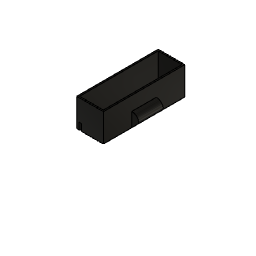
Seitenteil_links_Schublade_v56 (Autodesk Fusion 360 design; units mm, degrees)
Autodesk Fusion 360 part; units mm, degrees
sketch "Skizze1" plane through (70, 0, 0) normal (1, 0, 0) x (0, 1, 0)
  line L0 (59.1546, 143.1) -> (59.1546, 102.1)
  line L1 (59.1546, 102.1) -> (-58.1, 102.1)
  line L2 (-58.1, 102.1) -> (-58.1, 143.1)
  line L3 (-58.1, 143.1) -> (59.1546, 143.1)
  line L4 (-74.1, 83.1) -> (74.1, 83.1)
  line L5 (74.1, 83.1) -> (74.1, 152.2)
  arc A0 (74.1, 152.2) -> (73.2, 153.1) centre (73.2, 152.2) ccw
  line L6 (73.2, 153.1) -> (-73.2, 153.1)
  arc A1 (-73.2, 153.1) -> (-74.1, 152.2) centre (-73.2, 152.2) ccw
  line L7 (-74.1, 152.2) -> (-74.1, 83.1)
  line L8 (-58.1, 102.1) -> (-58.1, 143.1)
  line L9 (-58.1, 143.1) -> (59.1546, 143.1)
  line L10 (59.1546, 143.1) -> (59.1546, 102.1)
  line L11 (59.1546, 102.1) -> (-58.1, 102.1)
  line L12 (-57.6, 142.6) -> (58.6546, 142.6)
  line L13 (58.6546, 142.6) -> (58.6546, 102.6)
  line L14 (58.6546, 102.6) -> (-57.6, 102.6)
  line L15 (-57.6, 102.6) -> (-57.6, 142.6)
  dimension "d664" = 0.5
  dimension "d665" = 0.5
  dimension "d666" = 0.5
  dimension "d667" = 0.5
  constraint horizontal L12
  constraint vertical L13
  constraint horizontal L14
  constraint vertical L15
  measures "d664" distance of L8 L15
  measures "d665" distance of L10 L13
  measures "d666" distance of L9 L12
  measures "d667" distance of L11 L14
extrude "Extrusion1" add sketch "Skizze1" against normal blind 38 contours L12 L13 L14 L15
shell "Schale1" thickness 2 removed faces 1 at (57.3333, -18.8485, 142.6)
sketch "Skizze7" plane through (0, 0, 102.6) normal (0, 0, -1) x (1, 0, 0)
  line L0 (70, -58.6546) -> (70, 57.6)
  line L1 (70, 57.6) -> (32, 57.6)
  line L2 (32, 57.6) -> (32, -58.6546)
  line L3 (32, -58.6546) -> (70, -58.6546)
  circle A0 centre (37, 58.6) radius 2
  circle A1 centre (37, -59.6546) radius 2
  dimension "d728" = 4
  dimension "d730" = 33
  dimension "d731" = 4
  dimension "d749" = 1
  dimension "d750" = 1
  constraint vertical A0.centre A1.centre
  measures "d728" diameter of A0
  measures "d730" distance of L0 A0.centre
  measures "d731" diameter of A1
  measures "d749" distance of L3 A1.centre
  measures "d750" distance of L1 A0.centre
extrude "Extrusion4" cut sketch "Skizze7" against normal up to surface (9.5 mm away) contours L3 A1 | L1 A0 picked at (36.8035, -58.1862) picked at (37.4433, 57.1448)
ref_plane "Arbeitsebene2" through (51, 0.5273, 122.6) normal (0, 1, 0) x (0, 0, -1)
sketch "Skizze4" plane through (51, 0.5273, 124.1) normal (0, 1, 0) x (1, 0, 0)
  arc A0 (19, 1.5) -> (29, 11.5) centre (19, 11.5) ccw
  line L0 (19, -18.5) -> (19, 21.5)
  line L1 (29, 11.5) -> (19, 11.5)
  dimension "d709" = 10
  dimension "d710" = 10
  constraint vertical A0.centre L0.end
  constraint vertical A0.start L0.end
  constraint horizontal A0.centre A0.end
  constraint coincident A0.centre L1.end
  measures "d709" radius of A0
  measures "d710" distance of A0.centre L0.end
extrude "Extrusion2" add sketch "Skizze4" along normal mid plane 35
chamfer "Fase2" distance 10 angle 45 1 edges at (70, 0.5273, 112.6)
sketch "Skizze6" plane through (51, 0.5273, 124.1) normal (0, 1, 0) x (1, 0, 0)
  arc A0 (19, 1.5) -> (29, 11.5) centre (19, 11.5) ccw
  line L0 (19, 21.5) -> (19, 1.5)
  arc A1 (19, 1.5) -> (29, 11.5) centre (19, 11.5) ccw
  line L1 (19, -28.1) -> (19, 41)
  arc A2 (19, 3) -> (27.5, 11.5) centre (18.3872, 12.1128) ccw
  line L2 (19, 3) -> (19, 11.5)
  line L3 (29, 11.5) -> (19, 21.5)
  line L4 (27.5, 11.5) -> (29, 11.5)
  line L5 (29, 11.5) -> (19, 21.5)
  line L6 (19, 11.5) -> (19, 21.5)
  dimension "d714" = 1.5
  dimension "d719" = 1.5
  constraint coincident L0 A2.start
  constraint horizontal A0.end A2.end
  constraint coincident A0.centre A1.centre
  constraint coincident A0.end A1.end
  constraint coincident L0.start L3.end
  constraint tangent A0 A2
  measures "d714" horizontal distance of A0.end A2.end
  measures "d719" distance of A0.start A2.start
extrude "Extrusion3" cut sketch "Skizze6" along normal mid plane 30 contours L0 L1 A2 L2 L3 L4 L5 L6
equation "d665 = d664"
equation "d666 = d664"
equation "d667 = d664"
equation "d714 = d713"
equation "d719 = d714"
equation "d713 = 1.5 mm"
